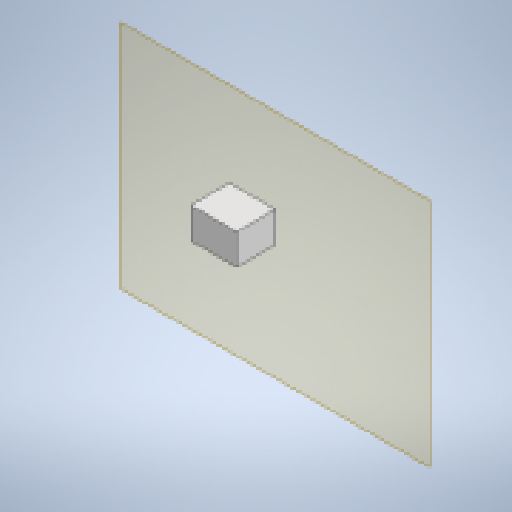
# Autodesk Inventor part: Mueble Acuario
Saved by Autodesk Inventor 2024 (Build 280153000, 153)
## iProperties
Created: 2024-04-05
Part Number: Mueble Acuario
Material: Genérico
Document SubType Name: Modeling
Designer: sergi
Density: 1 g/cm^3
Appearance: Valor por defecto
Author: sergi
Autodesk Inventor part; units mm, degrees
ref_plane "YZ Plane" through (0, 0, 0) normal (1, 0, 0) x (0, 1, 0)
ref_plane "XZ Plane" through (0, 0, 0) normal (0, 1, 0) x (-1, 0, 0)
ref_plane "XY Plane" through (0, 0, 0) normal (0, 0, 1) x (1, 0, 0)
ref_plane "Plano de trabajo1" through (54.7727, -256.5512, 0) normal (0, 0, 1) x (1, 0, 0)
sketch "Boceto1" plane through (54.7727, -256.5512, 0) normal (0, 0, 1) x (1, 0, 0)
  line L0 (-54.7727, 256.5512) -> (-954.7727, 256.5512)
  line L1 (-954.7727, 256.5512) -> (-954.7727, 656.5512)
  line L2 (-954.7727, 656.5512) -> (-54.7727, 656.5512)
  line L3 (-54.7727, 656.5512) -> (-54.7727, 256.5512)
  dimension "d0" = 900
  dimension "d1" = 400
  constraints: 8 end point, 2 parallel, 1 horizontal, 1 perpendicular
  measures "d0" distance of L1.end L2.end
  measures "d1" distance of L0.end L1.end
extrude "Extrusión1" add sketch "Boceto1" along normal blind 760
